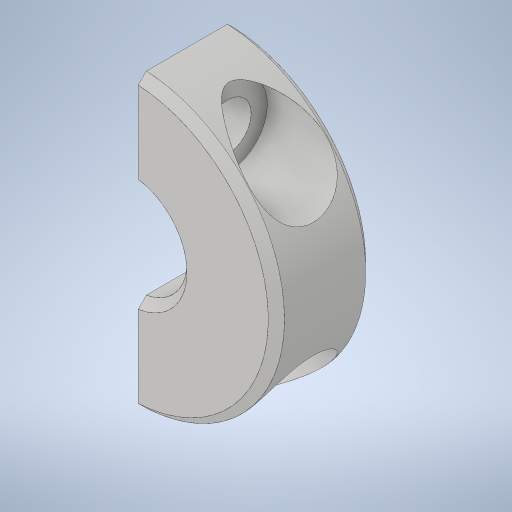
# Autodesk Inventor part: PSCSPJ6-6b
Saved by Autodesk Inventor 2024.1 (Build 281209000, 209)
## iProperties
Created: 2023-10-07
Part Number: PSCSPJ6-6b
Material: Generic
Catalog Web Link: www.cadenas.de
Description: SCSPJ, PSCSPJ, SSCSPJ, SCNPAJ, SCNPAWJ_b-Set Collars - Separate - Standard Compact Type
Vendor: MISUMI
Document SubType Name: Modeling
Designer: psAdmin
Manufacturer: MISUMI
Mass: 0.469199 g
Surface Area: 5.79924 cm^2
Volume: 0.469199 cm^3
Density: 1 g/cm^3
Appearance: PSOLRGB-191-191-191
Category: PARTsolutions
Company: MISUMI
PSOL_IDENT_0: {$CADENAS_DATA/23d-libs/misumi/metric/03_set_collars/scspj/scspj_b.prj},201 {VTYP=3D},{NB=PSCSPJ6-6b
PSOL_IDENT_1: },{LINA=PSCSPJ6-6b},{NN=SCSPJ, PSCSPJ, SSCSPJ, SCNPAJ, SCNPAWJ_b},{DATE=18.06.2021 05:26:24},{GEOMDA
PSOL_IDENT_2: TE=08.06.2021 05:07:29},{VERSION=},{LINEID=300},{WBVAR=MAT,ST},{WBNUMERIC=}  {NB=PSCSPJ6-6b},{LINA=P
PSOL_IDENT_3: SCSPJ6-6b},{KT=DUMMY},{PN=PSCSPJ6-6},{TYPE=PSCSPJ},{MAT=1},{MATALG='1','1045 Carbon Steel','2','SUS3
PSOL_IDENT_4: 04 Equivalent','3','2017 Aluminum Alloy'},{ST=2},{AC=Hexagon Socket Head Cap Screw 1 Pc. (SUS)},{D=6
PSOL_IDENT_5: },{B=6},{D1=18},{M=M2.6},{M1=2.6},{STALG='1','Black Oxide','2','Electroless Nickel Plating'},{DD=2.9
PSOL_IDENT_6: },{R=2.45},{W=1.0},{X=6.0},{Y=3.0},{C=0.5},{L=6},{COLOR=0.75,0.75,0.75,0.00},{LS=6}
NB: PSCSPJ6-6b
NN: SCSPJ, PSCSPJ, SSCSPJ, SCNPAJ, SCNPAWJ_b
NT: Set Collars - Separate - Standard Compact Type
NBSYN: $PN.b
LINA: PSCSPJ6-6b
CATALOG: Misumi
PN: PSCSPJ6-6
MAT: 1045 Carbon Steel
ST: Electroless Nickel Plating
AC: Hexagon Socket Head Cap Screw 1 Pc. (SUS)
D: 6
B: 6
D1: 18
M1: 2.6
DD: 2.9
R: 2.45
W: 1
X: 6
Y: 3
C: 0.5
L: 6
LS: 6
SUPPLIER: MISUMI
ARTICLENO: PSCSPJ6-6b
BOMINFO: PSCSPJ6-6b
CREATOR: CADENAS GmbH
Title: PSCSPJ6-6b
Author: Cadenas PARTsolutions
Comments: Set Collars - Separate - Standard Compact Type
Autodesk Inventor part; units mm, degrees
sketch "Sketch_1" plane through (0, 0, 0) normal (1, 0, 0) x (0, 1, 0)
  line L0 (0, -3) -> (0, 3)
  line L1 (8.5, 3) -> (3.5, 3)
  line L2 (3.5, 3) -> (3, 2.5)
  line L3 (3, 2.5) -> (3, -2.5)
  line L4 (3, -2.5) -> (3.5, -3)
  line L5 (3.5, -3) -> (8.5, -3)
  line L6 (8.5, -3) -> (9, -2.5)
  line L7 (9, -2.5) -> (9, 2.5)
  line L8 (9, 2.5) -> (8.5, 3)
  constraints: 18 end point
revolve "Revolution1" add sketch "Sketch_1" angle 180 about axis through (0, 0, -3) along (0, 0, -1)
sketch "Sketch_2" plane through (0, 0, 0) normal (0, 0, 1) x (1, 0, 0)
  line L0 (-0.5, -9) -> (0.5, -9)
  line L1 (0.5, -9) -> (0.5, 9)
  line L2 (0.5, 9) -> (-0.5, 9)
  line L3 (-0.5, 9) -> (-0.5, -9)
  constraints: 8 end point
extrude "Extrusion1" cut sketch "Sketch_2" along normal mid plane 6
sketch "Sketch_3" plane through (0, 0, 0) normal (0, 0, 1) x (1, 0, 0)
  line L0 (9, -6) -> (0, -6)
  line L1 (0, -6) -> (0, -4.55)
  line L2 (0, -4.55) -> (3, -4.55)
  line L3 (3, -4.55) -> (3, -3.55)
  line L4 (3, -3.55) -> (9, -3.55)
  line L5 (9, -3.55) -> (9, -6)
  line L6 (9, -6) -> (0, -6)
  constraints: 14 end point
revolve "Revolution2" cut sketch "Sketch_3" angle 360 about axis through (9, -6, 0) along (-1, 0, 0)
sketch "Sketch_4" plane through (0, 0, 0) normal (0, 0, 1) x (1, 0, 0)
  line L0 (9, 6) -> (0, 6)
  line L1 (0, 6) -> (0, 7.45)
  line L2 (0, 7.45) -> (3, 7.45)
  line L3 (3, 7.45) -> (3, 8.45)
  line L4 (3, 8.45) -> (9, 8.45)
  line L5 (9, 8.45) -> (9, 6)
  line L6 (9, 6) -> (0, 6)
  constraints: 14 end point
revolve "Revolution3" cut sketch "Sketch_4" angle 360 about axis through (9, 6, 0) along (-1, 0, 0)
ref_plane "1_2_XY" through (0, 0, 0) normal (1, 0, 0) x (0, 0, -1)
ref_plane "1_2_YZ" through (0, 0, 0) normal (0, 0, -1) x (0, 1, 0)
ref_plane "1_2_ZX" through (0, 0, 0) normal (0, 1, 0) x (1, 0, 0)
ref_plane "body_screw_XY" through (3, -6, 0) normal (1, 0, 0) x (0, 0, -1)
ref_plane "body_screw_YZ" through (3, -6, 0) normal (0, 0, -1) x (0, 1, 0)
ref_plane "body_screw_ZX" through (3, -6, 0) normal (0, 1, 0) x (1, 0, 0)
ref_plane "body_screw2_XY" through (3, 6, 0) normal (1, 0, 0) x (0, 0, -1)
ref_plane "body_screw2_YZ" through (3, 6, 0) normal (0, 0, -1) x (0, 1, 0)
ref_plane "body_screw2_ZX" through (3, 6, 0) normal (0, 1, 0) x (1, 0, 0)
body "Solid1"
